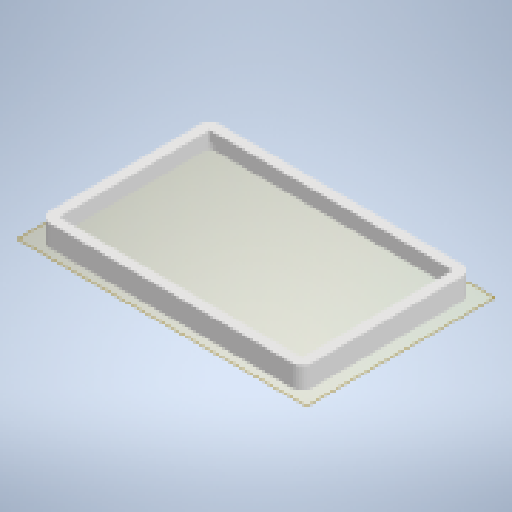
# Autodesk Inventor part: Gehaeuse_oben
Saved by Autodesk Inventor 2024 (Build 280153000, 153)
## iProperties
Created: 2025-04-09
Part Number: Gehaeuse_oben
Material: Generisch
Document SubType Name: Modeling
Designer: erikt
Density: 1 g/cm^3
Appearance: Vorgabe
Author: erikt
Autodesk Inventor part; units mm, degrees
ref_plane "YZ Plane" through (0, 0, 0) normal (1, 0, 0) x (0, 1, 0)
ref_plane "XZ Plane" through (0, 0, 0) normal (0, 1, 0) x (-1, 0, 0)
ref_plane "XY Plane" through (0, 0, 0) normal (0, 0, 1) x (1, 0, 0)
ref_plane "Arbeitsebene1" through (0, 0, 0) normal (0, 0, 1) x (1, 0, 0)
sketch "Skizze1" plane through (0, 0, 0) normal (0, 0, 1) x (1, 0, 0)
  arc A0 (-23.82, 16.765) -> (-25.82, 14.765) centre (-23.82, 14.765) ccw projected
  line L0 (-25.82, -14.765) -> (-25.82, 14.765) projected
  arc A1 (-25.82, -14.765) -> (-23.82, -16.765) centre (-23.82, -14.765) ccw projected
  line L1 (23.82, -16.765) -> (-23.82, -16.765) projected
  arc A2 (23.82, -16.765) -> (25.82, -14.765) centre (23.82, -14.765) ccw projected
  line L2 (25.82, 14.765) -> (25.82, -14.765) projected
  arc A3 (25.82, 14.765) -> (23.82, 16.765) centre (23.82, 14.765) ccw projected
  line L3 (-23.82, 16.765) -> (23.82, 16.765) projected
  arc A4 (23.82, -15.765) -> (24.82, -14.765) centre (23.82, -14.765) ccw projected
  line L4 (-23.82, -15.765) -> (23.82, -15.765) projected
  arc A5 (-24.82, -14.765) -> (-23.82, -15.765) centre (-23.82, -14.765) ccw projected
  line L5 (-24.82, 14.765) -> (-24.82, -14.765) projected
  arc A6 (-23.82, 15.765) -> (-24.82, 14.765) centre (-23.82, 14.765) ccw projected
  line L6 (23.82, 15.765) -> (-23.82, 15.765) projected
  arc A7 (24.82, 14.765) -> (23.82, 15.765) centre (23.82, 14.765) ccw projected
  line L7 (24.82, -14.765) -> (24.82, 14.765) projected
  arc A8 (-23.82, 15.965) -> (-25.02, 14.765) centre (-23.82, 14.765) ccw
  line L8 (-25.02, 14.765) -> (-25.02, -14.765)
  arc A9 (-25.02, -14.765) -> (-23.82, -15.965) centre (-23.82, -14.765) ccw
  line L9 (-23.82, -15.965) -> (23.82, -15.965)
  arc A10 (23.82, -15.965) -> (25.02, -14.765) centre (23.82, -14.765) ccw
  line L10 (25.02, -14.765) -> (25.02, 14.765)
  arc A11 (25.02, 14.765) -> (23.82, 15.965) centre (23.82, 14.765) ccw
  line L11 (23.82, 15.965) -> (-23.82, 15.965)
  point P0 (0, 0)
  dimension "d0" = 0.2
  constraints: 8 end point, 8 point on circle, 4 centre point, 7 other
  measures "d0" distance between parallel lines of L6 L11
extrude "Extrusion1" add sketch "Skizze1" along normal blind 2.2 contours L3 A3 L2 A2 L1 A1 L0 A0
sketch "Skizze2" plane through (0, 0, 2.2) normal (0, 0, 1) x (1, 0, 0)
  line L0 (23.82, 16.765) -> (-23.82, 16.765) projected
  line L1 (23.82, 14.765) -> (-23.82, 14.765) projected
  arc A0 (-24.82, -14.765) -> (-23.82, -15.765) centre (-23.82, -14.765) ccw projected
  line L2 (-23.82, -15.765) -> (23.82, -15.765) projected
  arc A1 (23.82, -15.765) -> (24.82, -14.765) centre (23.82, -14.765) ccw projected
  line L3 (24.82, -14.765) -> (24.82, 14.765) projected
  arc A2 (24.82, 14.765) -> (23.82, 15.765) centre (23.82, 14.765) ccw projected
  line L4 (23.82, 15.765) -> (-23.82, 15.765) projected
  arc A3 (-23.82, 15.765) -> (-24.82, 14.765) centre (-23.82, 14.765) ccw projected
  line L5 (-24.82, 14.765) -> (-24.82, -14.765) projected
  line L6 (-23.82, 14.765) -> (-23.82, -14.765) projected
  line L7 (23.82, 14.765) -> (-23.82, 14.765) projected
  line L8 (23.82, -14.765) -> (23.82, 14.765) projected
  line L9 (-23.82, -14.765) -> (23.82, -14.765) projected
  line L10 (23.82, 16.765) -> (-23.82, 16.765) projected
  arc A4 (-23.82, 16.765) -> (-25.82, 14.765) centre (-23.82, 14.765) ccw projected
  line L11 (-25.82, 14.765) -> (-25.82, -14.765) projected
  arc A5 (-25.82, -14.765) -> (-23.82, -16.765) centre (-23.82, -14.765) ccw projected
  line L12 (-23.82, -16.765) -> (23.82, -16.765) projected
  arc A6 (23.82, -16.765) -> (25.82, -14.765) centre (23.82, -14.765) ccw projected
  line L13 (25.82, -14.765) -> (25.82, 14.765) projected
  arc A7 (25.82, 14.765) -> (23.82, 16.765) centre (23.82, 14.765) ccw projected
  line L14 (-23.82, 15.965) -> (23.82, 15.965) projected
  arc A8 (25.02, 14.765) -> (23.82, 15.965) centre (23.82, 14.765) ccw projected
  line L15 (25.02, 14.765) -> (25.02, -14.765) projected
  arc A9 (23.82, -15.965) -> (25.02, -14.765) centre (23.82, -14.765) ccw projected
  line L16 (23.82, -15.965) -> (-23.82, -15.965) projected
  arc A10 (-25.02, -14.765) -> (-23.82, -15.965) centre (-23.82, -14.765) ccw projected
  line L17 (-25.02, -14.765) -> (-25.02, 14.765) projected
  arc A11 (-23.82, 15.965) -> (-25.02, 14.765) centre (-23.82, 14.765) ccw projected
  point P0 (0, 0)
extrude "Extrusion2" add sketch "Skizze2" along normal blind 38 contours A7 L13 A6 L12 A5 L11 A4 L0 | L5 A3 L4 A2 L3 A1 L2 A0 | L14 A8 L15 A9 L16 A10 L17 A11
sketch "Skizze3" plane through (-23.82, -16.765, 0) normal (0, -1, 0) x (1, 0, 0)
  line L0 (-2, 0) -> (-2, 40.2) projected
  line L1 (0, 40.2) -> (-2, 40.2) projected
  line L2 (0, 40.2) -> (47.64, 40.2) projected
  line L3 (49.64, 0) -> (49.64, 40.2) projected
  line L4 (49.64, 40.2) -> (47.64, 40.2) projected
  line L5 (49.64, 0) -> (47.64, 0) projected
  line L6 (0, 0) -> (47.64, 0) projected
  line L7 (-2, 0) -> (0, 0) projected
  line L8 (5.82, 38.2) -> (41.82, 38.2)
  line L9 (41.82, 38.2) -> (41.82, 4.2)
  line L10 (41.82, 4.2) -> (5.82, 4.2)
  line L11 (5.82, 4.2) -> (5.82, 38.2)
  point P0 (23.82, 0)
  dimension "d5" = 36
  dimension "d6" = 34
  dimension "d7" = 2
  dimension "d8" = 7.82
  dimension "d9" = 7.82
  constraints: 8 end point, 2 parallel, 1 horizontal, 1 perpendicular
  measures "d5" distance of L9.end L10.end
  measures "d6" distance of L8.end L9.end
  measures "d7" distance between parallel lines of L2 L8
  measures "d8" distance between parallel lines of L11 L0
  measures "d9" distance between parallel lines of L3 L9
extrude "Extrusion3" cut sketch "Skizze3" against normal up to surface (2 mm away) contours L8 L9 L10 L11
sketch "Skizze4" plane through (-23.82, -16.765, 0) normal (0, -1, 0) x (1, 0, 0)
  line L0 (5.82, 4.2) -> (5.82, 38.2) projected
  line L1 (5.82, 4.2) -> (5.82, 38.2) projected
  line L2 (5.82, 38.2) -> (41.82, 38.2) projected
  line L3 (41.82, 38.2) -> (41.82, 4.2) projected
  line L4 (41.82, 4.2) -> (5.82, 4.2) projected
  line L5 (0, 0) -> (47.64, 0) projected
  line L6 (47.64, 0) -> (47.64, 40.2) projected
  line L7 (0, 40.2) -> (47.64, 40.2) projected
  line L8 (0, 0) -> (0, 40.2) projected
  line L9 (42.02, 38.4) -> (5.62, 38.4)
  line L10 (5.62, 38.4) -> (5.62, 4)
  line L11 (5.62, 4) -> (42.02, 4)
  line L12 (42.02, 4) -> (42.02, 38.4)
  point P0 (23.82, 0)
  dimension "d12" = 0.2
  constraints: 8 end point, 3 other
  measures "d12" distance between parallel lines of L2 L9
extrude "Extrusion4" cut sketch "Skizze4" against normal up to surface (2 mm away) contours L12 L11 L10 L9
sketch "Skizze5" plane through (-23.82, -16.765, 0) normal (0, -1, 0) x (1, 0, 0)
  line L0 (5.62, 38.4) -> (42.02, 38.4) projected
  line L1 (42.02, 38.4) -> (42.02, 4) projected
  line L2 (42.02, 4) -> (5.62, 4) projected
  line L3 (5.62, 4) -> (5.62, 38.4) projected
  line L4 (0, 0) -> (47.64, 0) projected
  line L5 (47.64, 0) -> (47.64, 40.2) projected
  line L6 (0, 40.2) -> (47.64, 40.2) projected
  line L7 (0, 0) -> (0, 40.2) projected
  line L8 (31.32, 4.2) -> (31.32, 9.2) projected
  line L9 (31.32, 4.2) -> (41.82, 4.2) projected
  line L10 (41.82, 4.2) -> (41.82, 38.2) projected
  line L11 (41.82, 38.2) -> (5.82, 38.2) projected
  line L12 (5.82, 38.2) -> (5.82, 4.2) projected
  line L13 (5.82, 4.2) -> (16.32, 4.2) projected
  line L14 (16.32, 9.2) -> (16.32, 4.2) projected
  line L15 (31.32, 9.2) -> (16.32, 9.2) projected
  line L16 (40.82, 32.4) -> (6.82, 32.4) projected
  line L17 (40.82, 9.4) -> (40.82, 32.4) projected
  line L18 (6.82, 9.4) -> (40.82, 9.4) projected
  line L19 (6.82, 32.4) -> (6.82, 9.4) projected
  circle A0 centre (39.2325, 35.4875) radius 2.0875 projected
  circle A1 centre (8.4075, 35.4875) radius 2.0875 projected
  circle A2 centre (8.4075, 6.9125) radius 2.0875 projected
  circle A3 centre (39.2325, 6.9125) radius 2.0875 projected
  line L20 (28.63, 35.95) -> (26.63, 35.95) projected
  line L21 (26.63, 35.95) -> (26.63, 37.95) projected
  line L22 (26.63, 37.95) -> (28.63, 37.95) projected
  line L23 (28.63, 37.95) -> (28.63, 35.95) projected
  line L24 (26.09, 35.95) -> (24.09, 35.95) projected
  line L25 (24.09, 35.95) -> (24.09, 37.95) projected
  line L26 (24.09, 37.95) -> (26.09, 37.95) projected
  line L27 (26.09, 37.95) -> (26.09, 35.95) projected
  line L28 (21.55, 35.95) -> (21.55, 37.95) projected
  line L29 (21.55, 37.95) -> (23.55, 37.95) projected
  line L30 (23.55, 37.95) -> (23.55, 35.95) projected
  line L31 (23.55, 35.95) -> (21.55, 35.95) projected
  line L32 (19.01, 37.95) -> (21.01, 37.95) projected
  line L33 (21.01, 37.95) -> (21.01, 35.95) projected
  line L34 (21.01, 35.95) -> (19.01, 35.95) projected
  line L35 (19.01, 35.95) -> (19.01, 37.95) projected
  line L36 (6.62, 32.6) -> (41.02, 32.6)
  line L37 (41.02, 32.6) -> (41.02, 9.2)
  line L38 (41.02, 9.2) -> (6.62, 9.2)
  line L39 (6.62, 9.2) -> (6.62, 32.6)
  line L40 (19.01, 35.95) -> (28.63, 35.95)
  line L41 (28.63, 35.95) -> (28.63, 37.95)
  line L42 (28.63, 37.95) -> (19.01, 37.95)
  line L43 (19.01, 37.95) -> (19.01, 35.95)
  line L44 (29.13, 35.45) -> (18.51, 35.45)
  line L45 (18.51, 35.45) -> (18.51, 38.45)
  line L46 (18.51, 38.45) -> (29.13, 38.45)
  line L47 (29.13, 38.45) -> (29.13, 35.45)
  line L48 (16.02, 4.5) -> (6.12, 4.5)
  line L49 (6.12, 4.5) -> (6.12, 37.9)
  line L50 (6.12, 37.9) -> (41.52, 37.9)
  line L51 (41.52, 37.9) -> (41.52, 4.5)
  line L52 (41.52, 4.5) -> (31.62, 4.5)
  line L53 (31.62, 4.5) -> (31.62, 9.5)
  line L54 (31.62, 9.5) -> (16.02, 9.5)
  line L55 (16.02, 9.5) -> (16.02, 4.5)
  line L56 (16.02, 4.5) -> (16.02, 4)
  line L57 (31.62, 4.5) -> (31.62, 4)
  point P0 (23.82, 0)
  dimension "d15" = 0.2
  dimension "d16" = 0.5
  dimension "d17" = 0.3
  constraints: 44 end point, 4 parallel, 4 perpendicular, 2 point on line, 1 horizontal, 13 other
  measures "d15" distance between parallel lines of L16 L36
  measures "d16" distance between parallel lines of L40 L44
  measures "d17" distance between parallel lines of L14 L55
equation "\"d8\" = d9"
